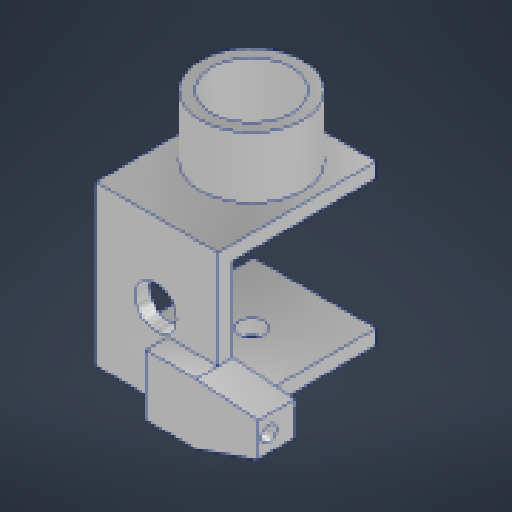
# Autodesk Inventor part: C23[i3][L]
Saved by Autodesk Inventor 2024 (Build 280153000, 153)
## iProperties
Created: 2020-12-02
Part Number: C23[i3][L]
Material: Aluminum 6061
Document SubType Name: Modeling
Designer: 57317
Density: 2.7 g/cm^3
Appearance: Aluminum - Flat
Author: 57317
Autodesk Inventor part; units mm, degrees
ref_plane "YZ Plane" through (0, 0, 0) normal (1, 0, 0) x (0, 1, 0)
ref_plane "XZ Plane" through (0, 0, 0) normal (0, 1, 0) x (-1, 0, 0)
ref_plane "XY Plane" through (0, 0, 0) normal (0, 0, 1) x (1, 0, 0)
sketch "Sketch1" plane through (0, 0, 0) normal (0, 0, 1) x (1, 0, 0)
  line L0 (25.5, -27) -> (-25.5, -27)
  line L1 (-25.5, -27) -> (-25.5, 27)
  line L2 (-25.5, 27) -> (25.5, 27)
  line L3 (25.5, 27) -> (25.5, -27)
  line L4 (25.5, -27) -> (-25.5, 27) construction
  line L5 (-25.5, -27) -> (25.5, 27) construction
  point P0 (0, 0)
  dimension "d0" = 51
  dimension "d1" = 54
  constraints: 12 end point, 2 midpoint, 2 parallel, 1 horizontal, 1 perpendicular
  measures "d0" distance of L1.end L2.end
  measures "d1" distance of L0.end L1.end
extrude "Extrusion1" add sketch "Sketch1" along normal blind 6
sketch "Sketch2" plane through (0, 0, 6) normal (0, 0, 1) x (1, 0, 0)
  circle A0 centre (0, 0) radius 15
  dimension "d4" = 30
  constraints: 1 centre point, 1 coincident
  measures "d4" diameter of A0
sketch "Sketch4" plane through (0, 0, 6) normal (0, 0, 1) x (1, 0, 0)
  line L0 (-25.5, 27) -> (26.5, 27)
  line L1 (-25.5, -27) -> (25.5, -27) projected
  line L2 (25.5, -27) -> (-25.5, -27)
  line L3 (-25.5, -27) -> (-25.5, -33)
  line L4 (-25.5, -33) -> (25.5, -33)
  line L5 (25.5, -33) -> (25.5, -27)
  point P0 (0, 0)
  dimension "d109" = 51
  dimension "d110" = 6
  constraints: 10 end point, 2 horizontal, 2 parallel, 1 perpendicular
  measures "d109" distance of L4.end L3.end
  measures "d110" distance of L3.end L2.end
extrude "Extrusion4" add sketch "Sketch4" against normal blind 65.3
ref_plane "Plano de trabajo8" through (25.5, -33.8, -42) normal (1, 0, 0) x (0, 0, -1)
ref_plane "Work Plane9" through (-10.5, -27, -57) normal (0, 1, 0) x (1, 0, 0)
sketch "Sketch25" plane through (-10.5, -27, -57) normal (0, 1, 0) x (1, 0, 0)
  line L0 (0, 0) -> (21, 0) projected
  line L1 (10.5, 0) -> (10.5, -23)
  circle A0 centre (10.5, -23) radius 5
  line L2 (10.5, -23) -> (10.5, -63)
  line L3 (36, -63) -> (-15, -63) projected
  point P0 (10.5, -57)
  dimension "d111" = 23
  dimension "d112" = 10
  constraints: 4 end point, 2 midpoint, 1 centre point, 1 coincident, 1 vertical
  measures "d111" distance of L1.start L1.end
  measures "d112" diameter of A0
extrude "Extrusion22" cut sketch "Sketch25" against normal blind 68
ref_plane "Work Plane7" through (-10.5, -0.5, -57) normal (0, 1, 0) x (1, 0, 0)
mirror "Mirror2" about plane through (-10.5, -0.5, -57) normal (0, 1, 0) of "Extrusion4"
extrude "Extrusión28" cut sketch "Sketch2" against normal blind 10
ref_plane "Work Plane10" through (25.5, -34, -42) normal (1, 0, 0) x (0, 0, -1)
ref_plane "Work Plane11" through (-25.5, -87, 1.3) normal (0, 1, 0) x (1, 0, 0)
sketch "Sketch37" plane through (-25.5, 32, 6) normal (0, 1, 0) x (1, 0, 0)
  circle A0 centre (25.5, 40) radius 5 projected
  point P0 (25.5, 6)
extrude "Extrusion33" cut sketch "Sketch37" against normal blind 68
sketch "Sketch43" plane through (0, 0, 6) normal (0, 0, 1) x (1, 0, 0)
  circle A0 centre (0, 0) radius 10.4895
  circle A1 centre (0, 0) radius 15 projected
  circle A2 centre (0, 0) radius 5
  dimension "d182" = 10
  constraints: 2 centre point, 2 coincident
  measures "d182" diameter of A2
extrude "Extrusion40" add sketch "Sketch43" against normal blind 8.3 contours A0 | A1
sketch "Boceto48" plane through (-25.5, -33, 6) normal (0, -1, 0) x (1, 0, 0)
  point P0 (25.5, -6)
sketch "Boceto49" plane through (-25.5, -33, 6) normal (0, -1, 0) x (1, 0, 0)
  point P0 (25.5, -6)
sketch "Boceto50" plane through (25.5, 26, -59.3) normal (0, 0, -1) x (-1, 0, 0)
  point P0 (25.5, -26)
sketch "Boceto77" plane through (0, 0, 6) normal (0, 0, 1) x (1, 0, 0)
  point P0 (0, 0)
sketch "Boceto84" plane through (25.5, -33, -59.3) normal (1, 0, 0) x (0, 0, -1)
  line L0 (-65.3, 0) -> (-65.3, 65) projected
  line L1 (-65.3, 0) -> (-65.3, 32.3804)
  line L2 (-65.3, 32.3804) -> (-80.5662, 32.3804)
  line L3 (-80.5662, 32.3804) -> (-80.5662, -6.9517)
  line L4 (-80.5662, -6.9517) -> (-65.3, -6.9517)
  line L5 (-65.3, -6.9517) -> (-65.3, 0)
  point P0 (-59.3, 33)
  point P1 (-65.3, 66.9563)
  point P2 (-65.3, 65.9563)
  constraints: 10 end point, 2 perpendicular, 2 point on line, 1 horizontal
extrude "Extrusión80" cut sketch "Boceto84" along normal mid plane 100
sketch "Boceto85" plane through (0, 0, 0) normal (0, 0, -1) x (-1, 0, 0)
  line L0 (-25.5, -33) -> (-25.5, -4.0448)
  line L1 (-25.5, -27) -> (-25.5, 26) projected
  line L2 (-25.5, -4.0448) -> (-53.9802, -4.6672)
  line L3 (-53.9802, -4.6672) -> (-54.6281, -33.6366)
  line L4 (-54.6281, -33.6366) -> (-25.5, -33)
  point P0 (0, 0)
  point P1 (-25.5, -13.7947)
  constraints: 8 end point, 1 parallel, 1 point on line
extrude "Extrusión81" cut sketch "Boceto85" along normal mid plane 100
sketch "Boceto90" plane through (0, 0, 6) normal (0, 0, 1) x (1, 0, 0)
  circle A0 centre (0, 0) radius 5.2249
  circle A1 centre (0, 0) radius 14.4421
  constraints: 2 centre point, 2 coincident
extrude "Extrusión86" add sketch "Boceto90" along normal blind 4.7
fillet "Empalme20" radius 2 1 edges at (-14.4421, 0, 6)
sketch "Boceto91" plane through (0, 0, 0) normal (0, 0, -1) x (-1, 0, 0)
  point P0 (0, 0)
sketch "Boceto92" plane through (0, 0, 0) normal (0, 0, -1) x (-1, 0, 0)
  point P0 (0, 0)
sketch "Boceto93" plane through (0, 0, 0) normal (0, 0, -1) x (-1, 0, 0)
  line L0 (-25.5, -27) -> (-25.5, 26) projected
  line L1 (-25.5, 1.3668) -> (-41.5813, 1.3668)
  line L2 (-41.5813, 1.3668) -> (-41.5813, -33)
  line L3 (-25.5, -33) -> (-41.5813, -33)
  line L4 (-25.5, -33) -> (-25.5, 32.9563) projected
  line L5 (-25.5, 1.3668) -> (-25.5, -33)
  point P0 (0, 0)
  constraints: 8 end point, 2 horizontal, 1 perpendicular, 1 point on line, 1 vertical
extrude "Extrusión87" add sketch "Boceto93" against normal blind 8.3
sketch "Boceto94" plane through (0, 0, 6) normal (0, 0, 1) x (1, 0, 0)
  line L0 (41.5813, -33) -> (41.5813, 1.3668) projected
  line L1 (41.5813, 1.3668) -> (41.5813, 35.5236)
  line L2 (-25.5, 32.9563) -> (25.5, 32.9563) projected
  line L3 (25.5, 32.9563) -> (41.5813, 32.9563)
  line L4 (25.5, 32.9563) -> (25.5, 1.3668)
  line L5 (25.5, 1.3668) -> (41.5813, 1.3668)
  point P0 (0, 0)
  constraints: 8 end point, 2 vertical, 1 collinear, 1 perpendicular, 1 point on line
extrude "Extrusión88" add sketch "Boceto94" against normal blind 8.3
sketch "Boceto95" plane through (0, 0, 6) normal (0, 0, 1) x (1, 0, 0)
  circle A0 centre (37.8913, -24.81) radius 2.6
  line L0 (35.2913, -24.81) -> (37.8913, -24.81)
  point P0 (0, 0)
  point P1 (41.5813, -33)
  dimension "d305" = 5.2
  constraints: 2 end point, 1 centre point, 1 horizontal
  measures "d305" diameter of A0
extrude "Extrusión89" cut sketch "Boceto95" against normal blind 8.3
sketch "Boceto97" plane through (-25.5, -33, -59.3) normal (-1, 0, 0) x (0, 0, 1)
  line L0 (59.3, 0) -> (67.6, 0) projected
  line L1 (67.6, 0) -> (89.1392, 0)
  line L2 (89.1392, 0) -> (89.1392, 69.8717)
  line L3 (89.1392, 69.8717) -> (67.6, 69.8717)
  line L4 (67.6, 69.8717) -> (67.6, 0)
  point P0 (59.3, 33)
  constraints: 8 end point, 2 parallel, 1 horizontal, 1 perpendicular
extrude "Extrusión92" cut sketch "Boceto97" against normal blind 1000
sketch "Boceto98" plane through (-25.5, -33, -59.3) normal (-1, 0, 0) x (0, 0, 1)
  line L0 (59.3, 59) -> (59.3, 6) projected
  line L1 (59.3, 59) -> (58.3, 59) projected
  line L2 (59.3, 6) -> (59.3, 59)
  line L3 (59.3, 59) -> (56.1979, 59)
  line L4 (59.3, 59) -> (0, 59) projected
  line L5 (56.1979, 59) -> (56.1979, 6)
  line L6 (59.3, 6) -> (0, 6) projected
  line L7 (56.1979, 6) -> (59.3, 6)
  line L8 (65.3, 65) -> (0, 65) projected
  line L9 (56.1979, 65) -> (56.1979, 67.4992)
  line L10 (56.1979, 67.4992) -> (67.7631, 67.4992)
  line L11 (67.7631, 67.4992) -> (76.364, 67.4992)
  line L12 (76.364, 67.4992) -> (76.364, -7.6447)
  line L13 (65.3, 0) -> (65.3, 34.3668) projected
  line L14 (65.3, 0) -> (65.3, -7.6447)
  line L15 (65.3, -7.6447) -> (76.364, -7.6447)
  line L16 (65.3, 0) -> (65.3, 65)
  line L17 (65.3, 0) -> (65.3, 65) projected
  line L18 (56.1979, 65) -> (65.3, 65)
  point P0 (59.3, 33)
  point P1 (59.3, 51.8098)
  point P2 (58.3, 65)
  point P3 (65.3, 65.9563)
  point P4 (59.3, 51.8098)
  point P5 (58.3, 65)
  point P6 (65.3, 34.3668)
  constraints: 25 end point, 4 perpendicular, 4 vertical, 3 point on line, 1 collinear
extrude "Extrusión93" cut sketch "Boceto98" along normal mid plane 1000
sketch "Boceto99" plane through (41.5813, -33, 0) normal (1, 0, 0) x (0, 0, -1)
  line L0 (0, 58.9816) -> (2.3, 58.9816)
  line L1 (2.3, 65) -> (2.3, 59) projected
  line L2 (2.3, 58.9816) -> (2.3, 65)
  line L3 (2.3, 65) -> (2.3, 58.9816)
  line L4 (2.3, 65) -> (0, 65)
  line L5 (-6, 65) -> (59.3, 65) projected
  line L6 (0, 58.9816) -> (0, 65)
  point P0 (0, 33)
  constraints: 10 end point, 2 perpendicular, 1 collinear, 1 horizontal, 1 point on line
extrude "Extrusión94" cut sketch "Boceto99" against normal blind 16.081
sketch "Boceto100" plane through (25.5, 26, -59.3) normal (0, 0, -1) x (-1, 0, 0)
  line L0 (-16.0813, 6) -> (-0.0003, 6) projected
  line L1 (0, 0) -> (-16.0813, 0)
  line L2 (-16.0813, 0) -> (-16.0813, 6)
  line L3 (-16.0813, 6) -> (0, 6)
  line L4 (0, 6) -> (0, 0)
  point P0 (25.5, -26)
  point P1 (-0.0003, 6)
  constraints: 8 end point, 2 parallel, 1 horizontal, 1 perpendicular
extrude "Extrusión95" cut sketch "Boceto100" against normal blind 59.3
sketch "Boceto101" plane through (0, 0, 0) normal (0, 0, -1) x (-1, 0, 0)
  circle A0 centre (0, 0) radius 8.5
  dimension "d322" = 17
  constraints: 1 centre point, 1 coincident
  measures "d322" diameter of A0
extrude "Extrusión96" cut sketch "Boceto101" against normal blind 59.3
sketch "Boceto102" plane through (-25.5, 32, -59.3) normal (0, 1, 0) x (1, 0, 0)
  circle A0 centre (25.5, -25.3) radius 5 projected
  circle A1 centre (25.5, -25.3) radius 16.3
  circle A2 centre (25.5, -25.3) radius 21
  point P0 (25.5, -59.3)
  dimension "d325" = 32.6
  dimension "d326" = 42
  constraints: 2 centre point, 2 coincident
  measures "d325" diameter of A1
  measures "d326" diameter of A2
extrude "Extrusión97" add sketch "Boceto102" along normal blind 25 contours A2
sketch "Boceto103" plane through (-25.5, -27, -59.3) normal (0, 1, 0) x (1, 0, 0)
  point P0 (25.5, -59.3)
sketch "Boceto104" plane through (0, 0, 6) normal (0, 0, 1) x (1, 0, 0)
  line L0 (-25.5, -33) -> (-25.5, 32) projected
  line L1 (41.5813, 32) -> (41.5813, -33) projected
  line L2 (-25.5, 32) -> (41.5813, 32)
  line L3 (41.5813, 32) -> (41.5813, -33)
  line L4 (41.5813, -33) -> (-25.5, -33)
  line L5 (-25.5, -33) -> (-25.5, 32)
  point P0 (0, 0)
  constraints: 8 end point, 2 parallel, 1 horizontal, 1 perpendicular
extrude "Extrusión98" cut sketch "Boceto104" against normal blind 0.8
sketch "Boceto105" plane through (0, 0, 0) normal (0, 0, -1) x (-1, 0, 0)
  line L0 (-25.5, -33) -> (25.5, -33) projected
  line L1 (-41.5813, 32) -> (25.5, 32)
  line L2 (25.5, 32) -> (25.5, -33)
  line L3 (25.5, -33) -> (-41.5813, -33)
  line L4 (-41.5813, -33) -> (-41.5813, 32)
  circle A0 centre (-37.8913, -24.81) radius 2.6 projected
  circle A1 centre (-37.8913, -24.81) radius 2.6
  circle A2 centre (0, 0) radius 8.5
  constraints: 8 end point, 2 centre point, 2 coincident, 2 parallel, 1 horizontal, 1 perpendicular
extrude "Extrusión99" add sketch "Boceto105" along normal blind 0.8
sketch "Boceto106" plane through (-25.5, -33, -59.3) normal (0, -1, 0) x (1, 0, 0)
  line L0 (0, 0) -> (51, 0) projected
  line L1 (67.0813, 64.5) -> (0, 64.5) projected
  line L2 (0, 0) -> (1, 0)
  line L3 (1, 0) -> (1, 64.5)
  line L4 (1, 64.5) -> (0, 64.5)
  line L5 (0, 64.5) -> (0, 0)
  point P0 (25.5, 59.3)
  point P1 (0, 64.5)
  point P2 (1, 0)
  dimension "d333" = 1
  constraints: 8 end point, 2 parallel, 1 horizontal, 1 perpendicular, 1 point on line
  measures "d333" distance of L4.end L3.end
extrude "Extrusión100" cut sketch "Boceto106" against normal blind 1000
sketch "Boceto107" plane through (0, 0, -0.8) normal (0, 0, -1) x (-1, 0, 0)
  line L0 (-25.5, -33) -> (-25.5, -38.9196)
  line L1 (-25.5, -38.9196) -> (-33.0828, -52.767)
  line L2 (-33.0828, -52.767) -> (-34.3078, -45.7968) construction
  line L3 (-41.5813, -33) -> (24.5, -33) projected
  spline S0 degree 3 poles (-33.0828, -52.767) (-34.3078, -45.7968) (-36.0426, -41.6296) (-38.17, -38.0712) knots 1 1 1 1 1.670244 1.670244 1.670244 1.670244
  line L4 (-41.5813, 32) -> (-41.5813, -33) projected
  line L5 (-37.8729, -38.2076) -> (-46.4829, -34.2556)
  line L6 (-46.4829, -34.2556) -> (-46.4829, 32)
  line L7 (-46.4829, 32) -> (-41.5813, 32)
  line L8 (-34.3078, -45.7968) -> (-36.0426, -41.6296) construction
  line L9 (-36.0426, -41.6296) -> (-38.17, -38.0712) construction
  point P0 (0, 0)
  constraints: 10 end point, 1 parallel, 1 perpendicular, 1 point on line, 1 vertical, 3 other
extrude "Extrusión101" add sketch "Boceto107" against normal blind 6
fillet "Empalme21" radius 2 2 edges at (38.17, -38.0712, 2.2) (46.4829, -34.2556, 2.2)
sketch "Boceto108" plane through (-24.5, -33, 5.2) normal (0, -1, 0) x (1, 0, 0)
  circle A0 centre (24.5, -39.2) radius 5 projected
  line L0 (24.5, -39.2) -> (24.5, -15.2)
  line L1 (50, -6) -> (0, -6) projected
  line L2 (24.5, -15.2) -> (32.2045, -6)
  line L3 (32.2045, -6) -> (24.5, -15.2)
  line L4 (24.5, -15.2) -> (36.5, -15.2)
  line L5 (36.5, -15.2) -> (12.5, -15.2)
  circle A1 centre (36.5, -15.2) radius 5.975
  circle A2 centre (12.5, -15.2) radius 5.975
  point P0 (24.5, -5.2)
  dimension "d340" = 24
  dimension "d341" = 12
  dimension "d342" = 12
  dimension "d343" = 24
  dimension "d344" = 11.95
  dimension "d345" = 11.95
  constraints: 10 end point, 2 centre point, 2 coincident, 2 perpendicular, 2 point on line, 1 collinear
  measures "d340" distance of L0.start L0.end
  measures "d341" distance of L0.end L2.end
  measures "d342" distance of L0.end L4.end
  measures "d343" distance of L4.end L5.end
  measures "d344" diameter of A1
  measures "d345" diameter of A2
extrude "Extrusión102" add sketch "Boceto108" along normal blind 2.5 contours A1 | A2
sketch "Boceto109" plane through (0, 0, -0.8) normal (0, 0, -1) x (-1, 0, 0)
  line L0 (-45.3172, -34.7906) -> (-38.7421, -37.8086) projected
  line L1 (-45.3172, -34.7906) -> (-49.6596, -32.7974)
  line L2 (-49.6596, -32.7974) -> (-49.6596, 32)
  line L3 (-46.4829, 32) -> (-46.4829, -32.9729) projected
  line L4 (-49.6596, 32) -> (-46.4829, 32)
  arc A0 (-46.4829, -32.9729) -> (-45.3172, -34.7906) centre (-44.4829, -32.9729) ccw projected
  line L5 (-46.4829, 32) -> (-45.3172, -34.7906)
  point P0 (0, 0)
  constraints: 8 end point, 1 collinear, 1 parallel, 1 perpendicular
extrude "Extrusión103" add sketch "Boceto109" against normal blind 6 contours L1 L2 L4 L3 A0
fillet "Empalme23" radius 4 2 edges at (49.6596, -32.7974, 2.2) (49.6596, 32, 2.2)
sketch "Boceto110" plane through (0, 0, 5.2) normal (0, 0, 1) x (1, 0, 0)
  line L0 (33.0828, -52.767) -> (25.5, -38.9196) projected
  line L1 (25.5, -38.9196) -> (37.9157, -38.9196)
  line L2 (37.9157, -38.9196) -> (33.0828, -52.767)
  line L3 (33.0828, -52.767) -> (25.5, -38.9196)
  point P0 (0, 0)
  constraints: 6 end point, 1 collinear, 1 horizontal
extrude "Extrusión104" cut sketch "Boceto110" against normal blind 10
sketch "Sketch111" plane through (0, 0, 5.2) normal (0, 0, 1) x (1, 0, 0)
  line L0 (25.5, -33) -> (25.5, -38.9196) projected
  line L1 (38.7421, -37.8086) -> (47.3283, -33.8675) projected
  line L2 (25.5, -33) -> (47.3283, -33.8675)
  line L3 (37.6774, -38.9196) -> (25.5, -38.9196) projected
  line L4 (25.5, -38.9196) -> (37.6774, -38.9196)
  line L5 (37.6774, -38.9196) -> (38.7421, -37.8086)
  point P0 (0, 0)
  constraints: 6 end point, 1 horizontal
extrude "Extrusion105" cut sketch "Sketch111" against normal blind 10
sketch "Sketch114" plane through (0, 0, -0.8) normal (0, 0, -1) x (-1, 0, 0)
  line L0 (-25.5, 32) -> (-25.5, 26) projected
  line L1 (-25.5, 26) -> (-25.5, 32)
  line L2 (-25.5, 32) -> (-25.5, -13.2226)
  line L3 (-25.5, -13.2226) -> (-49.6596, -13.2226)
  line L4 (-49.6596, -30.2322) -> (-49.6596, 28) projected
  line L5 (-49.6596, 28) -> (-49.6596, -30.2322) projected
  line L6 (-49.6596, -13.2226) -> (-49.6596, 28)
  line L7 (-25.5, 32) -> (-45.6596, 32) projected
  arc A0 (-45.6596, 32) -> (-49.6596, 28) centre (-45.6596, 28) ccw projected
  arc A1 (-45.6596, 32) -> (-49.6596, 28) centre (-45.6596, 28) ccw
  line L8 (-45.6596, 32) -> (-25.5, 32)
  point P0 (0, 0)
  constraints: 10 end point, 2 collinear, 2 point on circle, 2 point on line, 1 centre point, 1 concentric, 1 horizontal, 1 perpendicular
extrude "Extrusion108" cut sketch "Sketch114" against normal blind 6
sketch "Sketch115" plane through (0, 0, -59.3) normal (0, 0, -1) x (-1, 0, 0)
  line L0 (-50.9952, -38.1245) -> (29.0048, -38.1245)
  line L1 (29.0048, -38.1245) -> (29.0048, 81.8755)
  line L2 (29.0048, 81.8755) -> (-50.9952, 81.8755)
  line L3 (-50.9952, 81.8755) -> (-50.9952, -38.1245)
  point P0 (0, 0)
  dimension "d363" = 80
  dimension "d364" = 120
  constraints: 8 end point, 2 parallel, 1 horizontal, 1 perpendicular
  measures "d363" distance of L2.end L1.end
  measures "d364" distance of L1.end L0.end
sketch "Sketch116" plane through (0, 0, 5.2) normal (0, 0, 1) x (1, 0, 0)
  line L0 (25.5, -33) -> (-24.5, -33) projected
  line L1 (25.5, -33) -> (50.5194, -24.1438)
  line L2 (50.5194, -24.1438) -> (50.8592, -10.1321)
  line L3 (50.8592, -10.1321) -> (25.5, -8.1902)
  line L4 (25.5, 26) -> (25.5, -13.2226) projected
  line L5 (25.5, -27) -> (25.5, -33) projected
  line L6 (25.5, -33) -> (25.5, -8.1902)
  line L7 (25.5, -33) -> (62.3665, -33)
  line L8 (62.3665, -33) -> (62.3665, 19.7655)
  line L9 (62.3665, 19.7655) -> (25.5, 19.7655)
  line L10 (25.5, 19.7655) -> (25.5, -33)
  line L11 (62.3665, 19.7655) -> (25.5, 19.7655)
  line L12 (25.5, 19.7655) -> (25.5, -84.5573)
  line L13 (25.5, -84.5573) -> (62.3665, -84.5573)
  line L14 (62.3665, -84.5573) -> (62.3665, 19.7655)
  point P0 (0, 0)
  constraints: 24 end point, 4 parallel, 2 horizontal, 2 perpendicular, 2 point on line, 1 collinear
extrude "Extrusion109" add sketch "Sketch116" along normal blind 9 and the other way blind 6 contours L5 L6 L4 L3 L2 L1
sketch "Sketch117" plane through (50.8592, -10.1321, 14.2) normal (0.9997061, -0.0242446, 0) x (0, 0, -1)
  line L0 (1.2948, -7.0247) -> (1.2483, -7.0247)
  line L1 (0, 1.3265) -> (0, -23.476) projected
  line L2 (0, -7.0247) -> (9, -7.0247)
  line L3 (9, -23.476) -> (9, 1.3265) projected
  line L4 (4.5, -7.0247) -> (4.5, -10.2314)
  line L5 (4.5, -10.2314) -> (1.2483, -7.0247)
  circle A0 centre (4.5, -7.0247) radius 3.2517
  point P0 (14.2, 8.896)
  constraints: 8 end point, 2 point on line, 1 coincident, 1 horizontal, 1 horizontal alignment, 1 midpoint, 1 vertical, 2 other
extrude "Extrusion110" cut sketch "Sketch117" against normal blind 20
extrude "Extrusion111" cut sketch "Sketch116" against normal blind 20 contours L1 L2 L3 L4 L9 L8 L7 | L7 L14 L13 L12
sketch "Sketch118" plane through (0, 0, 5.2) normal (0, 0, 1) x (1, 0, 0)
  line L0 (25.5, -8.1902) -> (25.5, 32) projected
  line L1 (5, -33) -> (-5, -33) projected
  line L2 (25.5, -8.1902) -> (5, -33)
  line L3 (5, -33) -> (25.5, -33)
  line L4 (25.5, -33) -> (25.5, -8.1902)
  line L5 (25.5, -8.1902) -> (5, -8.1902)
  line L6 (-24.5, -27) -> (-24.5, 26) projected
  line L7 (5, -8.1902) -> (5, -33)
  point P0 (0, 0)
  constraints: 10 end point, 2 perpendicular, 1 collinear
extrude "Extrusion112" add sketch "Sketch118" along normal blind 9
ref_plane "Work Plane3" through (-10.35, 26, -57) normal (0, 1, 0) x (1, 0, 0)
body "Solid1"
